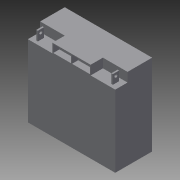
# Autodesk Inventor part: battery
Saved by Autodesk Inventor 2015 SP1 (Build 190203100, 203)
## iProperties
Created: 2014-10-23
Part Number: battery
Material: Generic
Document SubType Name: Modeling
Designer: 215152
Density: 1 g/cm^3
Appearance: Default
Author: 215152
Autodesk Inventor part; units mm, degrees
ref_plane "YZ Plane" through (0, 0, 0) normal (1, 0, 0) x (0, 1, 0)
ref_plane "XZ Plane" through (0, 0, 0) normal (0, 1, 0) x (-1, 0, 0)
ref_plane "XY Plane" through (0, 0, 0) normal (0, 0, 1) x (1, 0, 0)
sketch "Sketch1" plane through (0, 0, 0) normal (0, 1, 0) x (-1, 0, 0)
  line L0 (0, 0) -> (-180.34, 0)
  line L1 (-180.34, 0) -> (-180.34, -76.2)
  line L2 (-180.34, -76.2) -> (0, -76.2)
  line L3 (0, -76.2) -> (0, 0)
  dimension "d0" = 180.34
  dimension "d1" = 76.2
  constraints: 8 end point, 2 parallel, 1 horizontal, 1 perpendicular
  measures "d0" distance of L2.end L1.end
  measures "d1" distance of L1.end L0.end
extrude "Extrusion1" add sketch "Sketch1" along normal blind 167.64
sketch "Sketch2" plane through (0, 167.64, 0) normal (0, 1, 0) x (1, 0, 0)
  line L0 (0, 0) -> (180.34, 0) projected
  line L1 (180.34, 0) -> (180.34, 76.2) projected
  line L2 (180.34, 76.2) -> (0, 76.2) projected
  line L3 (0, 76.2) -> (0, 0) projected
  line L4 (0, 0) -> (50.8, 0)
  line L5 (50.8, 0) -> (50.8, 25.4)
  line L6 (50.8, 25.4) -> (0, 25.4)
  line L7 (0, 25.4) -> (0, 0)
  line L8 (180.34, 0) -> (129.54, 0)
  line L9 (129.54, 0) -> (129.54, 25.4)
  line L10 (129.54, 25.4) -> (180.34, 25.4)
  line L11 (180.34, 25.4) -> (180.34, 0)
  dimension "d4" = 50.8
  dimension "d5" = 25.4
  dimension "d6" = 50.8
  dimension "d7" = 25.4
  constraints: 16 end point, 4 parallel, 2 horizontal, 2 perpendicular
  measures "d4" distance of L6.end L5.end
  measures "d5" distance of L5.end L4.end
  measures "d6" distance of L9.end L10.end
  measures "d7" distance of L8.end L9.end
extrude "Extrusion2" cut sketch "Sketch2" against normal blind 19.05 contours L3 L6 L5 L0 | L9 L10 L1 L0
sketch "Sketch3" plane through (0, 0, 0) normal (0, 0, 1) x (1, 0, 0)
  line L0 (50.8, 167.64) -> (50.8, 148.59) construction
  line L1 (50.8, 148.59) -> (0, 148.59) projected
  line L2 (0, 0) -> (0, 148.59) projected
  line L3 (0, 0) -> (180.34, 0) projected
  line L4 (180.34, 0) -> (180.34, 148.59) projected
  line L5 (180.34, 148.59) -> (129.54, 148.59) projected
  line L6 (129.54, 148.59) -> (129.54, 167.64) construction
  line L7 (50.8, 167.64) -> (129.54, 167.64) construction
  line L8 (50.8, 167.64) -> (129.54, 167.64)
  line L9 (129.54, 167.64) -> (129.54, 148.59)
  line L10 (129.54, 148.59) -> (50.8, 148.59) construction
  line L11 (50.8, 148.59) -> (50.8, 167.64)
  line L12 (52.3875, 150.1775) -> (127.9525, 150.1775) construction
  line L13 (127.9525, 150.1775) -> (127.9525, 166.0525) construction
  line L14 (127.9525, 166.0525) -> (52.3875, 166.0525) construction
  line L15 (52.3875, 166.0525) -> (52.3875, 150.1775) construction
  line L16 (52.3875, 166.0525) -> (89.2175, 166.0525)
  line L17 (89.2175, 166.0525) -> (89.2175, 150.1775)
  line L18 (89.2175, 150.1775) -> (52.3875, 150.1775)
  line L19 (52.3875, 150.1775) -> (52.3875, 166.0525)
  line L20 (127.9525, 150.1775) -> (91.1225, 150.1775)
  line L21 (91.1225, 150.1775) -> (91.1225, 166.0525)
  line L22 (91.1225, 166.0525) -> (127.9525, 166.0525)
  line L23 (127.9525, 166.0525) -> (127.9525, 150.1775)
  dimension "d10" = 1.5875
  dimension "d11" = 36.83
  dimension "d12" = 36.83
  constraints: 32 end point, 8 parallel, 4 perpendicular, 3 horizontal, 2 point on line, 3 other
  measures "d10" distance between parallel lines of L10 L12
  measures "d11" distance of L17.end L18.end
  measures "d12" distance of L21.end L22.end
extrude "Extrusion3" cut sketch "Sketch3" against normal blind 12.7 contours L16 L17 L18 L19 | L20 L21 L22 L23
sketch "Sketch4" plane through (180.34, 0, -76.2) normal (0, 0, -1) x (-1, 0, 0)
  line L0 (0, 0) -> (180.34, 0) construction
  line L1 (180.34, 0) -> (180.34, 167.64) construction
  line L2 (0, 167.64) -> (180.34, 167.64) construction
  line L3 (0, 0) -> (0, 167.64) construction
  line L4 (0, 167.64) -> (180.34, 167.64) construction
  line L5 (180.34, 167.64) -> (180.34, 148.59) construction
  line L6 (180.34, 148.59) -> (0, 148.59) construction
  line L7 (0, 148.59) -> (0, 167.64) construction
  line L8 (1.5875, 150.1775) -> (178.7525, 150.1775) construction
  line L9 (178.7525, 150.1775) -> (178.7525, 166.0525) construction
  line L10 (178.7525, 166.0525) -> (1.5875, 166.0525) construction
  line L11 (1.5875, 166.0525) -> (1.5875, 150.1775) construction
  line L12 (1.5875, 166.0525) -> (44.5135, 166.0525)
  line L13 (44.5135, 166.0525) -> (44.5135, 150.1775)
  line L14 (44.5135, 150.1775) -> (1.5875, 150.1775)
  line L15 (1.5875, 150.1775) -> (1.5875, 166.0525)
  line L16 (178.7525, 150.1775) -> (135.8265, 150.1775)
  line L17 (135.8265, 150.1775) -> (135.8265, 166.0525)
  line L18 (135.8265, 166.0525) -> (178.7525, 166.0525)
  line L19 (178.7525, 166.0525) -> (178.7525, 150.1775)
  line L20 (46.101, 150.1775) -> (89.027, 150.1775)
  line L21 (89.027, 150.1775) -> (89.027, 166.0525)
  line L22 (89.027, 166.0525) -> (46.101, 166.0525)
  line L23 (46.101, 166.0525) -> (46.101, 150.1775)
  line L24 (134.239, 150.1775) -> (91.313, 150.1775)
  line L25 (91.313, 150.1775) -> (91.313, 166.0525)
  line L26 (91.313, 166.0525) -> (134.239, 166.0525)
  line L27 (134.239, 166.0525) -> (134.239, 150.1775)
  dimension "d15" = 1.5875
  dimension "d16" = 42.926
  dimension "d17" = 42.926
  dimension "d18" = 42.926
  dimension "d19" = 42.926
  dimension "d20" = 1.5875
  dimension "d21" = 1.5875
  constraints: 48 end point, 12 parallel, 6 perpendicular, 6 point on line, 5 horizontal, 3 other
  measures "d15" distance between parallel lines of L3 L11
  measures "d16" distance of L13.end L14.end
  measures "d17" distance of L17.end L18.end
  measures "d18" distance of L22.end L21.end
  measures "d19" distance of L25.end L26.end
  measures "d20" distance between parallel lines of L27 L17
  measures "d21" distance between parallel lines of L13 L23
extrude "Extrusion4" cut sketch "Sketch4" against normal blind 12.7
sketch "Sketch5" plane through (0, 148.59, 0) normal (0, 1, 0) x (1, 0, 0)
  line L0 (50.8, 0) -> (0, 0) projected
  line L1 (50.8, 25.4) -> (50.8, 0) projected
  line L2 (0, 25.4) -> (50.8, 25.4) projected
  line L3 (0, 0) -> (0, 25.4) projected
  line L4 (180.34, 25.4) -> (180.34, 0) projected
  line L5 (129.54, 25.4) -> (180.34, 25.4) projected
  line L6 (129.54, 0) -> (129.54, 25.4) projected
  line L7 (180.34, 0) -> (129.54, 0) projected
  line L8 (0, 0) -> (12.7, 0) construction
  line L9 (12.7, 0) -> (12.7, 12.7) construction
  line L10 (12.7, 12.7) -> (0, 12.7) construction
  line L11 (0, 12.7) -> (0, 0) construction
  line L12 (180.34, 0) -> (167.64, 0) construction
  line L13 (167.64, 0) -> (167.64, 12.7) construction
  line L14 (167.64, 12.7) -> (180.34, 12.7) construction
  line L15 (180.34, 12.7) -> (180.34, 0) construction
  line L16 (11.1125, 19.05) -> (14.2875, 19.05)
  line L17 (14.2875, 19.05) -> (14.2875, 6.35)
  line L18 (14.2875, 6.35) -> (11.1125, 6.35)
  line L19 (11.1125, 6.35) -> (11.1125, 19.05)
  line L20 (11.1125, 19.05) -> (14.2875, 6.35) construction
  line L21 (14.2875, 19.05) -> (11.1125, 6.35) construction
  line L22 (169.2275, 6.35) -> (166.0525, 6.35)
  line L23 (166.0525, 6.35) -> (166.0525, 19.05)
  line L24 (166.0525, 19.05) -> (169.2275, 19.05)
  line L25 (169.2275, 19.05) -> (169.2275, 6.35)
  line L26 (169.2275, 6.35) -> (166.0525, 19.05) construction
  line L27 (166.0525, 6.35) -> (169.2275, 19.05) construction
  dimension "d24" = 12.7
  dimension "d25" = 12.7
  dimension "d26" = 12.7
  dimension "d27" = 12.7
  dimension "d28" = 3.175
  dimension "d29" = 12.7
  dimension "d30" = 3.175
  dimension "d31" = 12.7
  constraints: 40 end point, 8 parallel, 4 horizontal, 4 midpoint, 4 perpendicular
  measures "d24" distance of L10.end L9.end
  measures "d25" distance of L9.end L8.end
  measures "d26" distance of L13.end L14.end
  measures "d27" distance of L12.end L13.end
  measures "d28" distance of L17.end L18.end
  measures "d29" distance of L16.end L17.end
  measures "d30" distance of L23.end L24.end
  measures "d31" distance of L22.end L23.end
extrude "Extrusion5" add sketch "Sketch5" along normal blind 19.05 contours L16 L17 L18 L19 | L22 L23 L24 L25
sketch "Sketch6" plane through (169.2275, 148.59, -6.35) normal (1, 0, 0) x (0, 0, -1)
  line L0 (12.7, 0) -> (0, 0) construction
  line L1 (12.7, 0) -> (12.7, 19.05) construction
  line L2 (0, 19.05) -> (12.7, 19.05) construction
  line L3 (0, 0) -> (0, 19.05) construction
  line L4 (0, 19.05) -> (6.35, 19.05) construction
  line L5 (6.35, 19.05) -> (6.35, 12.7) construction
  line L6 (6.35, 12.7) -> (0, 12.7) construction
  line L7 (0, 12.7) -> (0, 19.05) construction
  circle A0 centre (6.35, 12.7) radius 3.175
  point P0 (-6.35, -148.59)
  dimension "d34" = 6.35
  dimension "d35" = 6.35
  dimension "d36" = 6.35
  constraints: 8 end point, 2 parallel, 1 centre point, 1 coincident, 1 horizontal, 1 perpendicular
  measures "d34" distance of L5.end L6.end
  measures "d35" distance of L4.end L5.end
  measures "d36" diameter of A0
extrude "Extrusion6" cut sketch "Sketch6" against normal blind 25.4
sketch "Sketch7" plane through (11.1125, 148.59, -19.05) normal (-1, 0, 0) x (0, 0, 1)
  line L0 (12.7, 0) -> (0, 0) construction
  line L1 (12.7, 0) -> (12.7, 19.05) construction
  line L2 (0, 19.05) -> (12.7, 19.05) construction
  line L3 (0, 0) -> (0, 19.05) construction
  line L4 (12.7, 19.05) -> (6.35, 19.05) construction
  line L5 (6.35, 19.05) -> (6.35, 12.7) construction
  line L6 (6.35, 12.7) -> (12.7, 12.7) construction
  line L7 (12.7, 12.7) -> (12.7, 19.05) construction
  circle A0 centre (6.35, 12.7) radius 3.175
  point P0 (19.05, -148.59)
  dimension "d39" = 6.35
  dimension "d40" = 6.35
  dimension "d41" = 6.35
  constraints: 8 end point, 2 parallel, 1 centre point, 1 coincident, 1 horizontal, 1 perpendicular
  measures "d39" distance of L6.end L5.end
  measures "d40" distance of L5.end L4.end
  measures "d41" diameter of A0
extrude "Extrusion7" cut sketch "Sketch7" against normal blind 25.4
body "Solid1"
